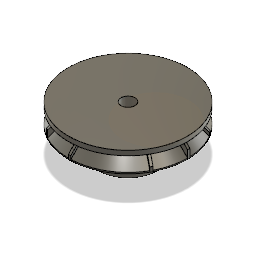
ropegear (Autodesk Fusion 360 design; units mm, degrees)
Autodesk Fusion 360 part; units mm, degrees
sketch "Sketch1" plane through (0, 0, 0) normal (0, 1, 0) x (1, 0, 0)
  circle A0 centre (0, 0) radius 12.5
  dimension "d1" = 25
  measures "d1" diameter of A0
extrude "Extrude1" add sketch "Sketch1" along normal blind 3 makes body 1
chamfer "Chamfer1" distance 3 angle 45 1 edges at (-11.6541, 3, 4.5202) on bodies 1
sketch "Sketch2" plane through (0, 3, 0) normal (0, 1, 0) x (-1, 0, 0)
  circle A0 centre (0, 0) radius 9.5
  circle A1 centre (0, 0) radius 12.5
  dimension "d5" = 25
  measures "d5" diameter of A1
extrude "Extrude2" add sketch "Sketch2" along normal blind 1 contours A0 | A1 bodies 1
sketch "Sketch3" plane through (0, 0, 0) normal (0, 0, 1) x (1, 0, 0)
  line L0 (0, 0) -> (0.5, 0)
  line L1 (0.5, 0) -> (0.5, 3)
  line L2 (0.5, 3) -> (0, 3)
  line L3 (0, 3) -> (0, 0)
  line L4 (12.5, 3) -> (-12.5, 3)
extrude "Extrude3" add sketch "Sketch3" along normal blind 12.5 separate body makes body 2
chamfer "Chamfer2" distance 2.3 angle 45 1 edges at (0.25, 3, 12.5) on bodies 2
pattern_circular "C-Pattern1" count 6 over 360 about axis through (0, 0, 0) along (0, 1, 0) of bodies 2 makes body 3 at (6.5529, 1, 3.7833) makes body 4 at (6.3029, 1, -4.2163) makes body 5 at (0, 1, -7.5667) makes body 6 at (-6.5529, 1, -3.7833) makes body 7 at (-6.5529, 1, 3.7833)
sketch "Sketch4" plane through (0, 0, 0) normal (0, 0, 1) x (1, 0, 0)
sketch "Sketch5" plane through (0, 0, 0) normal (1, 0, 0) x (0, 0, -1)
  line L0 (0, 0) -> (0.5, 0)
  line L1 (0.5, 0) -> (0.5, 3)
  line L2 (0.5, 3) -> (0, 3)
  line L3 (0, 3) -> (0, 0)
  line L4 (-0.433, 3) -> (4.667, 3)
extrude "Extrude4" add sketch "Sketch5" along normal blind 12.5 separate body makes body 8
chamfer "Chamfer3" distance 1.5 angle 45 1 edges at (12.5, 3, -0.25) on bodies 8
pattern_circular "C-Pattern2" count 3 over 360 about axis through (0, 0, 0) along (0, 1, 0) of bodies 8 makes body 9 at (-4.3497, 1, -6.5339) makes body 10 at (-3.9167, 1, 6.7839)
combine "Combine1" operation add target body 1 tool bodies 7 10 2 6 9 5 4 8 3
sketch "Sketch6" plane through (0, 0, 0) normal (0, -1, 0) x (1, 0, 0)
  arc A0 (10.8253, 6.25) -> (0.5, 12.49) centre (0, 0) ccw
  line L0 (0.5, 12.49) -> (0.5, 12.5)
  line L1 (0.5, 12.5) -> (0, 12.5)
  arc A1 (0, 12.5) -> (-5.812, 11.0667) centre (0, 0) ccw
  line L2 (-5.812, 11.0667) -> (-5.817, 11.0753)
  line L3 (-5.817, 11.0753) -> (-6.25, 10.8253)
  arc A2 (-6.25, 10.8253) -> (-10.5667, 6.678) centre (0, 0) ccw
  line L4 (-10.5667, 6.678) -> (-10.5753, 6.683)
  line L5 (-10.5753, 6.683) -> (-10.8253, 6.25)
  arc A3 (-10.8253, 6.25) -> (-11.0667, -5.812) centre (0, 0) ccw
  line L6 (-11.0667, -5.812) -> (-11.0753, -5.817)
  line L7 (-11.0753, -5.817) -> (-10.8253, -6.25)
  arc A4 (-10.8253, -6.25) -> (-6.678, -10.5667) centre (0, 0) ccw
  line L8 (-6.678, -10.5667) -> (-6.683, -10.5753)
  line L9 (-6.683, -10.5753) -> (-6.25, -10.8253)
  arc A5 (-6.25, -10.8253) -> (-0.5, -12.49) centre (0, 0) ccw
  line L10 (-0.5, -12.49) -> (-0.5, -12.5)
  line L11 (-0.5, -12.5) -> (0, -12.5)
  arc A6 (0, -12.5) -> (10.5667, -6.678) centre (0, 0) ccw
  line L12 (10.5667, -6.678) -> (10.5753, -6.683)
  line L13 (10.5753, -6.683) -> (10.8253, -6.25)
  arc A7 (10.8253, -6.25) -> (12.49, -0.5) centre (0, 0) ccw
  line L14 (12.49, -0.5) -> (12.5, -0.5)
  line L15 (12.5, -0.5) -> (12.5, 0)
  arc A8 (12.5, 0) -> (11.0667, 5.812) centre (0, 0) ccw
  line L16 (11.0667, 5.812) -> (11.0753, 5.817)
  line L17 (11.0753, 5.817) -> (10.8253, 6.25)
scale "Scale1" factor 1.8 about (7.9658, 3, -5.1764) bodies 1
sketch "Sketch7" plane through (0, -2.4, 0) normal (0, -1, 0) x (1, 0, 0)
  arc A0 (13.1129, 15.3911) -> (-5.4727, 26.6231) centre (-6.3727, 4.1411) ccw
  line L0 (-5.4727, 26.6231) -> (-5.4727, 26.6411)
  line L1 (-5.4727, 26.6411) -> (-6.3727, 26.6411)
  arc A1 (-6.3727, 26.6411) -> (-16.8342, 24.0611) centre (-6.3727, 4.1411) ccw
  line L2 (-16.8342, 24.0611) -> (-16.8432, 24.0767)
  line L3 (-16.8432, 24.0767) -> (-17.6227, 23.6267)
  arc A2 (-17.6227, 23.6267) -> (-25.3926, 16.1616) centre (-6.3727, 4.1411) ccw
  line L4 (-25.3926, 16.1616) -> (-25.4082, 16.1706)
  line L5 (-25.4082, 16.1706) -> (-25.8582, 15.3911)
  arc A3 (-25.8582, 15.3911) -> (-26.2926, -6.3204) centre (-6.3727, 4.1411) ccw
  line L6 (-26.2926, -6.3204) -> (-26.3082, -6.3294)
  line L7 (-26.3082, -6.3294) -> (-25.8582, -7.1089)
  arc A4 (-25.8582, -7.1089) -> (-18.3931, -14.8788) centre (-6.3727, 4.1411) ccw
  line L8 (-18.3931, -14.8788) -> (-18.4021, -14.8944)
  line L9 (-18.4021, -14.8944) -> (-17.6227, -15.3444)
  arc A5 (-17.6227, -15.3444) -> (-7.2727, -18.3408) centre (-6.3727, 4.1411) ccw
  line L10 (-7.2727, -18.3408) -> (-7.2727, -18.3589)
  line L11 (-7.2727, -18.3589) -> (-6.3727, -18.3589)
  arc A6 (-6.3727, -18.3589) -> (12.6473, -7.8793) centre (-6.3727, 4.1411) ccw
  line L12 (12.6473, -7.8793) -> (12.6629, -7.8883)
  line L13 (12.6629, -7.8883) -> (13.1129, -7.1089)
  arc A7 (13.1129, -7.1089) -> (16.1093, 3.2411) centre (-6.3727, 4.1411) ccw
  line L14 (16.1093, 3.2411) -> (16.1273, 3.2411)
  line L15 (16.1273, 3.2411) -> (16.1273, 4.1411)
  arc A8 (16.1273, 4.1411) -> (13.5473, 14.6027) centre (-6.3727, 4.1411) ccw
  line L16 (13.5473, 14.6027) -> (13.5629, 14.6117)
  line L17 (13.5629, 14.6117) -> (13.1129, 15.3911)
  circle A9 centre (-6.3727, 4.1411) radius 7.5
  dimension "d19" = 15
  measures "d19" diameter of A9
extrude "Extrude5" add sketch "Sketch7" along normal blind 10 contours A9 bodies 1
sketch "Sketch8" plane through (0, -12.4, 0) normal (0, -1, 0) x (1, 0, 0)
  circle A0 centre (-6.3727, 4.1411) radius 7.5
  circle A1 centre (-6.3727, 4.1411) radius 2.5
  dimension "d22" = 5
  measures "d22" diameter of A1
extrude "Extrude6" cut sketch "Sketch8" against normal blind 100 contours A1 bodies 1
sketch "Sketch9" plane through (0, 0, 0) normal (0, 0, 1) x (1, 0, 0)
  circle A0 centre (-6.3727, -6.4827) radius 1.375
  dimension "d25" = 2.75
  measures "d25" diameter of A0
extrude "Extrude7" add sketch "Sketch9" against normal blind 10 separate body makes body 11
move_body "Move1" bodies 11 to x (1, 0, 0) y (0, 1, 0) z (0, 0, 1) at (0, 0, 4)
combine "Combine2" operation cut target body 1 tool bodies 11
extrude "Extrude8" add 1 faces at (-5.1104, -2.4, -13.2744) along direction (0, -1, 0) blind 0.5 on bodies 1 bodies 1
move_face "OffsetFaces1" offset 3.5 1 faces at (-8.6648, -7.2979, -3) on bodies 1
move_face "OffsetFaces2" offset -0.13 1 faces at (-3.8851, -6.6667, 3.8922) on bodies 1
move_face "OffsetFaces3" offset -0.05 1 faces at (-5.2578, -5.6779, -3.9485) on bodies 1
sketch "Sketch10" plane through (0, 0, 0) normal (0, 0, 1) x (1, 0, 0)
  line L0 (-6.3727, -2.9) -> (12.6473, -2.9)
  line L1 (-3.4477, -6.4827) -> (-3.4477, -2.6827)
  line L2 (-9.2977, -6.4827) -> (-9.2977, -10.2827)
  line L3 (-9.2977, -10.2827) -> (-3.4477, -10.2827)
  line L4 (-3.4477, -10.2827) -> (-3.4477, -2.6827)
  line L5 (-3.4477, -2.6827) -> (-9.2977, -2.6827)
  line L6 (-9.2977, -2.6827) -> (-9.2977, -10.2827)
  dimension "d33" = 1.5
  dimension "d34" = 1.5
  dimension "d36" = 3.8
extrude "Extrude9" add sketch "Sketch10" against normal blind 3.4 separate body makes body 12
extrude "Extrude10" add 1 faces at (-7.3477, -10.2827, -1.1333) along direction (0, -1, 0) blind 5 on bodies 12 bodies 12
combine "Combine3" operation cut target body 1 tool bodies 12 keep tools
hidden bodies 12
